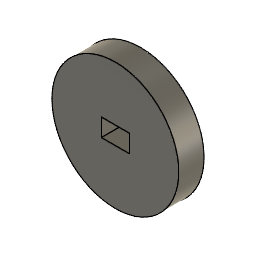
wheel-out (Autodesk Fusion 360 design; units mm, degrees)
Autodesk Fusion 360 part; units mm, degrees
sketch "Sketch1" plane through (0, 0, 0) normal (0, 1, 0) x (1, 0, 0)
  line L0 (1.2, -1) -> (-1.2, -1)
  line L1 (-1.2, -1) -> (-1.2, 1)
  line L2 (-1.2, 1) -> (1.2, 1)
  line L3 (1.2, 1) -> (1.2, -1)
  line L4 (1.2, -1) -> (-1.2, 1) construction
  line L5 (-1.2, -1) -> (1.2, 1) construction
  circle A0 centre (0, 0) radius 5
  dimension "d1" = 2.4
  dimension "d2" = 2
  constraint horizontal L0
  constraint perpendicular L0 L1
  constraint parallel L0 L2
  constraint parallel L1 L3
  constraint coincident L4 A0.centre
  constraint coincident L5 A0.centre
  constraint coincident A0.centre origin
  measures "d1" distance of L1.end L2.end
  measures "d2" distance of L0.end L1.end
extrude "Extrude1" add sketch "Sketch1" along normal blind 2
sketch "Sketch2" plane through (0, 0, 0) normal (0, -1, 0) x (1, 0, 0)
  line L0 (1.2, -1) -> (-1.2, -1)
  line L1 (-1.2, -1) -> (-1.2, 1)
  line L2 (-1.2, 1) -> (1.2, 1)
  line L3 (1.2, 1) -> (1.2, -1)
  circle A0 centre (0, 0) radius 5
  line L4 (1, 0.6) -> (-1, 0.6)
  line L5 (-1, 0.6) -> (-1, -0.6)
  line L6 (-1, -0.6) -> (1, -0.6)
  line L7 (1, -0.6) -> (1, 0.6)
  line L8 (1, 0.6) -> (-1, -0.6) construction
  line L9 (-1, 0.6) -> (1, -0.6) construction
  line L10 (-1.1, -0.7) -> (1.1, -0.7)
  line L11 (1.1, -0.7) -> (1.1, 0.7)
  line L12 (1.1, 0.7) -> (-1.1, 0.7)
  line L13 (-1.1, 0.7) -> (-1.1, -0.7)
  dimension "d5" = 2
  dimension "d6" = 1.2
  dimension "d7" = 0.1
  constraint horizontal L4
  constraint perpendicular L4 L5
  constraint parallel L4 L6
  constraint parallel L5 L7
  constraint coincident L8 A0.centre
  constraint coincident L9 A0.centre
  constraint coincident A0.centre origin
  measures "d5" distance of L5.end L6.end
  measures "d6" distance of L4.end L5.end
extrude "Extrude2" add sketch "Sketch2" against normal blind 2 contours L0 L1 L2 L3
